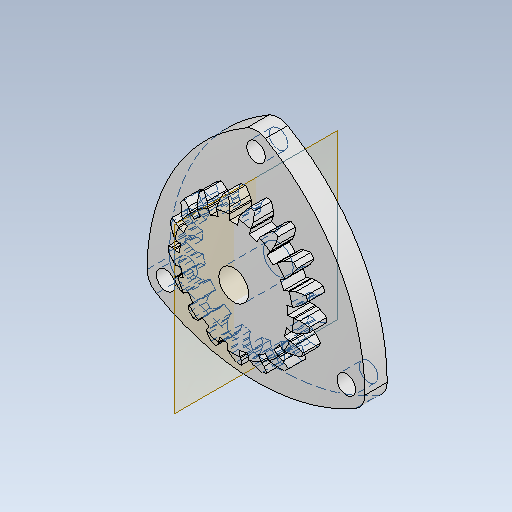
# Autodesk Inventor part: m1z17
Saved by Autodesk Inventor 2020 (Build 240168000, 168)
## iProperties
Created: 2020-10-28
Part Number: m1z17
Material: アルミニウム 2014-T4
Document SubType Name: Modeling
Designer: AA19065
Density: 2.8 g/cm^3
Appearance: サテン
Mass: 6.7317 g
Surface Area: 19.2727 cm^2
Volume: 2.40418 cm^3
Author: AA19065
Autodesk Inventor part; units mm, degrees
ref_plane "YZ Plane" through (0, 0, 0) normal (1, 0, 0) x (0, 1, 0)
ref_plane "XZ Plane" through (0, 0, 0) normal (0, 1, 0) x (-1, 0, 0)
ref_plane "XY Plane" through (0, 0, 0) normal (0, 0, 1) x (1, 0, 0)
sketch "スケッチ1" plane through (0, 0, 0) normal (0, 0, 1) x (1, 0, 0)
  arc A0 (149.1454, 113.0975) -> (149.1147, 112.9267) centre (149.977, 112.8598) ccw
  arc A1 (149.3297, 113.5561) -> (149.1454, 113.0975) centre (151.4433, 112.4406) ccw
  arc A2 (149.9133, 114.3943) -> (149.3297, 113.5561) centre (153.0232, 111.6068) ccw
  arc A3 (146.1768, 112.7838) -> (146.2098, 112.6135) centre (147.038, 112.8626) ccw
  arc A4 (146.1829, 113.2778) -> (146.1768, 112.7838) centre (148.5568, 113.0014) ccw
  arc A5 (146.4242, 114.2705) -> (146.1829, 113.2778) centre (150.3312, 112.7948) ccw
  arc A6 (143.5218, 111.419) -> (143.6141, 111.2721) centre (144.2964, 111.8035) ccw
  arc A7 (143.3491, 111.8818) -> (143.5218, 111.419) centre (145.6625, 112.4816) ccw
  arc A8 (143.2155, 112.8946) -> (143.3491, 111.8818) centre (147.3917, 112.93) ccw
  arc A9 (141.5392, 109.1872) -> (141.6783, 109.0836) centre (142.1226, 109.8256) ccw
  arc A10 (141.2109, 109.5563) -> (141.5392, 109.1872) centre (143.1514, 110.9514) ccw
  arc A11 (140.7205, 110.4525) -> (141.2109, 109.5563) centre (144.6019, 111.9941) ccw
  arc A12 (140.4967, 106.3899) -> (140.6638, 106.3435) centre (140.8101, 107.1959) ccw
  arc A13 (140.0572, 106.6155) -> (140.4967, 106.3899) centre (141.3627, 108.6174) ccw
  arc A14 (139.2762, 107.274) -> (140.0572, 106.6155) centre (142.3386, 110.1136) ccw
  arc A15 (140.535, 103.4049) -> (140.7076, 103.4221) centre (140.5361, 104.2697) ccw
  arc A16 (140.0437, 103.4565) -> (140.535, 103.4049) centre (140.538, 105.7948) ccw
  arc A17 (139.0776, 103.7885) -> (140.0437, 103.4565) centre (140.9074, 107.5426) ccw
  arc A18 (141.6491, 100.6353) -> (141.8039, 100.7137) centre (141.3377, 101.4421) ccw
  arc A19 (141.1723, 100.506) -> (141.6491, 100.6353) centre (140.7885, 102.8649) ccw
  arc A20 (140.1515, 100.4665) -> (141.1723, 100.506) centre (140.5016, 104.6281) ccw
  arc A21 (143.6884, 98.4552) -> (143.8044, 98.5842) centre (143.1066, 99.0951) ccw
  arc A22 (143.2906, 98.1624) -> (143.6884, 98.4552) centre (142.0805, 100.2234) ccw
  arc A23 (142.3529, 97.7568) -> (143.2906, 98.1624) centre (141.1761, 101.7639) ccw
  arc A24 (146.3776, 97.159) -> (146.4392, 97.3212) centre (145.6039, 97.5455) ccw
  arc A25 (146.1124, 96.7423) -> (146.3776, 97.159) centre (144.2395, 98.2269) ccw
  arc A26 (145.3846, 96.0254) -> (146.1124, 96.7423) centre (142.8397, 99.3367) ccw
  arc A27 (149.3534, 96.9218) -> (149.3522, 97.0953) centre (148.4924, 97.0027) ccw
  arc A28 (149.2566, 96.4374) -> (149.3534, 96.9218) centre (146.9739, 97.1453) ccw
  arc A29 (148.837, 95.506) -> (149.2566, 96.4374) centre (145.2677, 97.6744) ccw
  arc A30 (152.214, 97.7756) -> (152.1502, 97.9369) centre (151.3818, 97.54) ccw
  arc A31 (152.2987, 97.2889) -> (152.214, 97.7756) centre (149.9145, 97.1244) ccw
  arc A32 (152.2439, 96.2688) -> (152.2987, 97.2889) centre (148.1323, 97.0014) ccw
  arc A33 (154.5729, 99.6051) -> (154.4552, 99.7325) centre (153.8821, 99.0848) ccw
  arc A34 (154.8278, 99.1819) -> (154.5729, 99.6051) centre (152.6639, 98.1672) ccw
  arc A35 (155.1451, 98.2108) -> (154.8278, 99.1819) centre (151.0466, 97.4087) ccw
  arc A36 (156.1117, 102.1632) -> (155.9559, 102.2394) centre (155.6555, 101.4284) ccw
  arc A37 (156.5022, 101.8606) -> (156.1117, 102.1632) centre (154.8511, 100.1328) ccw
  arc A38 (157.1489, 101.0698) -> (156.5022, 101.8606) centre (153.6169, 98.8413) ccw
  arc A39 (156.6225, 105.1044) -> (156.4496, 105.1192) centre (156.4625, 104.2545) ccw
  arc A40 (157.0959, 104.9633) -> (156.6225, 105.1044) centre (156.1804, 102.7557) ccw
  arc A41 (157.9846, 104.4595) -> (157.0959, 104.9633) centre (155.4961, 101.1056) ccw
  arc A42 (156.0363, 108.0315) -> (155.8697, 107.9829) centre (156.1941, 107.1812) ccw
  arc A43 (156.5287, 108.071) -> (156.0363, 108.0315) centre (156.4725, 105.6818) ccw
  arc A44 (157.5394, 107.9223) -> (156.5287, 108.071) centre (156.4305, 103.8959) ccw
  arc A45 (154.4322, 110.5492) -> (154.2945, 110.4437) centre (154.8866, 109.8134) ccw
  arc A46 (154.8771, 110.7639) -> (154.4322, 110.5492) centre (155.6879, 108.5157) ccw
  arc A47 (155.8733, 110.9903) -> (154.8771, 110.7639) centre (156.2939, 106.8353) ccw
  arc A48 (152.027, 112.3175) -> (151.9367, 112.1693) centre (152.7165, 111.7954) ccw
  arc A49 (152.3643, 112.6784) -> (152.027, 112.3175) centre (153.9325, 110.8749) ccw
  arc A50 (153.2115, 113.2494) -> (152.3643, 112.6784) centre (155.1046, 109.5268) ccw
  arc A51 (147.8852, 112.9267) -> (147.8545, 113.0974) centre (147.023, 112.8598) ccw
  arc A52 (147.8545, 113.0974) -> (147.6704, 113.5559) centre (145.5566, 112.4406) ccw
  arc A53 (147.6704, 113.5559) -> (147.0867, 114.3943) centre (143.9767, 111.607) ccw
  arc A54 (145.0633, 112.1693) -> (144.973, 112.3175) centre (144.2835, 111.7954) ccw
  arc A55 (144.973, 112.3175) -> (144.6357, 112.6784) centre (143.0675, 110.8749) ccw
  arc A56 (144.6357, 112.6784) -> (143.7885, 113.2494) centre (141.8954, 109.5268) ccw
  arc A57 (142.7055, 110.4437) -> (142.5678, 110.5492) centre (142.1134, 109.8134) ccw
  arc A58 (142.5678, 110.5492) -> (142.1229, 110.7639) centre (141.3121, 108.5157) ccw
  arc A59 (142.1229, 110.7639) -> (141.1267, 110.9903) centre (140.7061, 106.8353) ccw
  arc A60 (141.1303, 107.9829) -> (140.9637, 108.0315) centre (140.8059, 107.1812) ccw
  arc A61 (140.9637, 108.0315) -> (140.4713, 108.071) centre (140.5275, 105.6818) ccw
  arc A62 (140.4713, 108.071) -> (139.4606, 107.9223) centre (140.5695, 103.8959) ccw
  arc A63 (140.5504, 105.1192) -> (140.3775, 105.1044) centre (140.5375, 104.2545) ccw
  arc A64 (140.3775, 105.1044) -> (139.9041, 104.9633) centre (140.8196, 102.7557) ccw
  arc A65 (139.9041, 104.9633) -> (139.0154, 104.4595) centre (141.5039, 101.1056) ccw
  arc A66 (141.0441, 102.2394) -> (140.8883, 102.1632) centre (141.3445, 101.4284) ccw
  arc A67 (140.8883, 102.1632) -> (140.4978, 101.8606) centre (142.1489, 100.1328) ccw
  arc A68 (140.4978, 101.8606) -> (139.8511, 101.0698) centre (143.3831, 98.8413) ccw
  arc A69 (142.5448, 99.7325) -> (142.4271, 99.6051) centre (143.1179, 99.0848) ccw
  arc A70 (142.4271, 99.6051) -> (142.1722, 99.1819) centre (144.3361, 98.1672) ccw
  arc A71 (142.1722, 99.1819) -> (141.8549, 98.2108) centre (145.9534, 97.4087) ccw
  arc A72 (144.8498, 97.9369) -> (144.786, 97.7756) centre (145.6182, 97.54) ccw
  arc A73 (144.786, 97.7756) -> (144.7013, 97.2889) centre (147.0855, 97.1244) ccw
  arc A74 (144.7013, 97.2889) -> (144.7561, 96.2688) centre (148.8677, 97.0014) ccw
  arc A75 (147.6478, 97.0953) -> (147.6466, 96.9218) centre (148.5076, 97.0027) ccw
  arc A76 (147.6466, 96.9218) -> (147.7434, 96.4374) centre (150.0261, 97.1453) ccw
  arc A77 (147.7434, 96.4374) -> (148.163, 95.506) centre (151.7323, 97.6744) ccw
  arc A78 (150.5608, 97.3212) -> (150.6224, 97.159) centre (151.3961, 97.5455) ccw
  arc A79 (150.6224, 97.159) -> (150.8876, 96.7423) centre (152.7605, 98.2269) ccw
  arc A80 (150.8876, 96.7423) -> (151.6154, 96.0254) centre (154.1603, 99.3367) ccw
  arc A81 (153.1956, 98.5842) -> (153.3116, 98.4552) centre (153.8934, 99.0951) ccw
  arc A82 (153.3116, 98.4552) -> (153.7094, 98.1624) centre (154.9195, 100.2234) ccw
  arc A83 (153.7094, 98.1624) -> (154.6471, 97.7568) centre (155.8239, 101.7639) ccw
  arc A84 (155.1961, 100.7137) -> (155.3509, 100.6353) centre (155.6623, 101.4421) ccw
  arc A85 (155.3509, 100.6353) -> (155.8277, 100.506) centre (156.2115, 102.8649) ccw
  arc A86 (155.8277, 100.506) -> (156.8485, 100.4665) centre (156.4984, 104.6281) ccw
  arc A87 (156.2924, 103.4221) -> (156.465, 103.4049) centre (156.4639, 104.2697) ccw
  arc A88 (156.465, 103.4049) -> (156.9563, 103.4565) centre (156.462, 105.7948) ccw
  arc A89 (156.9563, 103.4565) -> (157.9224, 103.7885) centre (156.0926, 107.5426) ccw
  arc A90 (156.3362, 106.3435) -> (156.5033, 106.3899) centre (156.1899, 107.1959) ccw
  arc A91 (156.5033, 106.3899) -> (156.9428, 106.6155) centre (155.6373, 108.6174) ccw
  arc A92 (156.9428, 106.6155) -> (157.7238, 107.274) centre (154.6614, 110.1136) ccw
  arc A93 (155.3217, 109.0836) -> (155.4608, 109.1872) centre (154.8774, 109.8256) ccw
  arc A94 (155.4608, 109.1872) -> (155.7891, 109.5563) centre (153.8486, 110.9514) ccw
  arc A95 (155.7891, 109.5563) -> (156.2795, 110.4525) centre (152.3981, 111.9941) ccw
  arc A96 (153.3859, 111.2721) -> (153.4782, 111.419) centre (152.7036, 111.8035) ccw
  arc A97 (153.4782, 111.419) -> (153.6509, 111.8818) centre (151.3375, 112.4816) ccw
  arc A98 (153.6509, 111.8818) -> (153.7845, 112.8946) centre (149.6083, 112.93) ccw
  arc A99 (150.7902, 112.6135) -> (150.8232, 112.7838) centre (149.962, 112.8626) ccw
  arc A100 (150.8232, 112.7838) -> (150.8171, 113.2778) centre (148.4432, 113.0014) ccw
  arc A101 (150.8171, 113.2778) -> (150.5758, 114.2705) centre (146.6688, 112.7948) ccw
  arc A102 (149.0605, 112.2283) -> (147.9394, 112.2283) centre (148.5, 105) ccw
  arc A103 (146.4115, 111.9427) -> (145.3661, 111.5377) centre (148.5, 105) ccw
  arc A104 (144.0446, 110.7194) -> (143.2161, 109.9641) centre (148.5, 105) ccw
  arc A105 (142.2793, 108.7237) -> (141.7796, 107.7201) centre (148.5, 105) ccw
  arc A106 (141.3543, 106.2251) -> (141.2508, 105.1088) centre (148.5, 105) ccw
  arc A107 (141.3942, 103.561) -> (141.701, 102.4827) centre (148.5, 105) ccw
  arc A108 (142.3939, 101.0913) -> (143.0695, 100.1966) centre (148.5, 105) ccw
  arc A109 (144.2182, 99.1495) -> (145.1714, 98.5593) centre (148.5, 105) ccw
  arc A110 (146.6208, 97.9978) -> (147.7228, 97.7918) centre (148.5, 105) ccw
  arc A111 (149.2772, 97.7918) -> (150.3792, 97.9978) centre (148.5, 105) ccw
  arc A112 (151.8286, 98.5593) -> (152.7818, 99.1495) centre (148.5, 105) ccw
  arc A113 (153.9305, 100.1966) -> (154.6061, 101.0913) centre (148.5, 105) ccw
  arc A114 (155.299, 102.4827) -> (155.6058, 103.561) centre (148.5, 105) ccw
  arc A115 (155.7492, 105.1088) -> (155.6457, 106.2251) centre (148.5, 105) ccw
  arc A116 (155.2204, 107.7201) -> (154.7207, 108.7237) centre (148.5, 105) ccw
  arc A117 (153.7839, 109.9641) -> (152.9554, 110.7194) centre (148.5, 105) ccw
  arc A118 (151.6339, 111.5377) -> (150.5885, 111.9427) centre (148.5, 105) ccw
  arc A119 (147.0867, 114.3943) -> (146.4242, 114.2705) centre (148.5, 105) ccw
  arc A120 (143.7885, 113.2494) -> (143.2155, 112.8946) centre (148.5, 105) ccw
  arc A121 (141.1267, 110.9903) -> (140.7205, 110.4525) centre (148.5, 105) ccw
  arc A122 (139.4606, 107.9223) -> (139.2762, 107.274) centre (148.5, 105) ccw
  arc A123 (139.0154, 104.4595) -> (139.0776, 103.7885) centre (148.5, 105) ccw
  arc A124 (139.8511, 101.0698) -> (140.1515, 100.4665) centre (148.5, 105) ccw
  arc A125 (141.8549, 98.2108) -> (142.3529, 97.7568) centre (148.5, 105) ccw
  arc A126 (144.7561, 96.2688) -> (145.3846, 96.0254) centre (148.5, 105) ccw
  arc A127 (148.163, 95.506) -> (148.837, 95.506) centre (148.5, 105) ccw
  arc A128 (151.6154, 96.0254) -> (152.2439, 96.2688) centre (148.5, 105) ccw
  arc A129 (154.6471, 97.7568) -> (155.1451, 98.2108) centre (148.5, 105) ccw
  arc A130 (156.8485, 100.4665) -> (157.1489, 101.0698) centre (148.5, 105) ccw
  arc A131 (157.9224, 103.7885) -> (157.9846, 104.4595) centre (148.5, 105) ccw
  arc A132 (157.7238, 107.274) -> (157.5394, 107.9223) centre (148.5, 105) ccw
  arc A133 (156.2795, 110.4525) -> (155.8733, 110.9903) centre (148.5, 105) ccw
  arc A134 (153.7845, 112.8946) -> (153.2115, 113.2494) centre (148.5, 105) ccw
  arc A135 (150.5758, 114.2705) -> (149.9133, 114.3943) centre (148.5, 105) ccw
  line L0 (149.0605, 112.2283) -> (149.1147, 112.9267)
  line L1 (146.4115, 111.9427) -> (146.2098, 112.6135)
  line L2 (144.0446, 110.7194) -> (143.6141, 111.2721)
  line L3 (142.2793, 108.7237) -> (141.6783, 109.0836)
  line L4 (141.3543, 106.2251) -> (140.6638, 106.3435)
  line L5 (141.3942, 103.561) -> (140.7076, 103.4221)
  line L6 (142.3939, 101.0913) -> (141.8039, 100.7137)
  line L7 (144.2182, 99.1495) -> (143.8044, 98.5842)
  line L8 (146.6208, 97.9978) -> (146.4392, 97.3212)
  line L9 (149.2772, 97.7918) -> (149.3522, 97.0953)
  line L10 (151.8286, 98.5593) -> (152.1502, 97.9369)
  line L11 (153.9305, 100.1966) -> (154.4552, 99.7325)
  line L12 (155.299, 102.4827) -> (155.9559, 102.2394)
  line L13 (155.7492, 105.1088) -> (156.4496, 105.1192)
  line L14 (155.2204, 107.7201) -> (155.8697, 107.9829)
  line L15 (153.7839, 109.9641) -> (154.2945, 110.4437)
  line L16 (151.6339, 111.5377) -> (151.9367, 112.1693)
  line L17 (147.9394, 112.2283) -> (147.8852, 112.9267)
  line L18 (145.3661, 111.5377) -> (145.0633, 112.1693)
  line L19 (143.2161, 109.9641) -> (142.7055, 110.4437)
  line L20 (141.7796, 107.7201) -> (141.1303, 107.9829)
  line L21 (141.2508, 105.1088) -> (140.5504, 105.1192)
  line L22 (141.701, 102.4827) -> (141.0441, 102.2394)
  line L23 (143.0695, 100.1966) -> (142.5448, 99.7325)
  line L24 (145.1714, 98.5593) -> (144.8498, 97.9369)
  line L25 (147.7228, 97.7918) -> (147.6478, 97.0953)
  line L26 (150.3792, 97.9978) -> (150.5608, 97.3212)
  line L27 (152.7818, 99.1495) -> (153.1956, 98.5842)
  line L28 (154.6061, 101.0913) -> (155.1961, 100.7137)
  line L29 (155.6058, 103.561) -> (156.2924, 103.4221)
  line L30 (155.6457, 106.2251) -> (156.3362, 106.3435)
  line L31 (154.7207, 108.7237) -> (155.3217, 109.0836)
  line L32 (152.9554, 110.7194) -> (153.3859, 111.2721)
  line L33 (150.5885, 111.9427) -> (150.7902, 112.6135)
  line L34 (137, 105) -> (160, 105)
  line L35 (148.5, 93.5) -> (148.5, 116.5)
  line L36 (178, 114.5) -> (248, 114.5)
  line L37 (178, 106.5) -> (248, 106.5)
  line L38 (178, 98.5) -> (248, 98.5)
  line L39 (178, 90.5) -> (248, 90.5)
  line L40 (178, 82.5) -> (248, 82.5)
  line L41 (178, 74.5) -> (248, 74.5)
  line L42 (178, 66.5) -> (248, 66.5)
  line L43 (178, 58.5) -> (248, 58.5)
  line L44 (178, 50.5) -> (248, 50.5)
  line L45 (178, 42.5) -> (248, 42.5)
  line L46 (178, 34.5) -> (248, 34.5)
  line L47 (178, 26.5) -> (248, 26.5)
  line L48 (178, 18.5) -> (248, 18.5)
  line L49 (178, 114.5) -> (178, 18.5)
  line L50 (248, 114.5) -> (248, 18.5)
  line L51 (213, 106.5) -> (213, 18.5)
  circle A136 centre (148.5, 105) radius 2
  circle A137 centre (148.5, 119) radius 1.25
  circle A138 centre (136.3756, 98) radius 1.25
  circle A139 centre (160.6244, 98) radius 1.25
  circle A140 centre (148.5, 119) radius 2.5
  circle A141 centre (136.3756, 98) radius 2.5
  circle A142 centre (160.6244, 98) radius 2.5
  arc A143 (147.25, 121.1651) -> (133.8756, 98) centre (160.6244, 98) ccw
  arc A144 (135.1256, 95.8349) -> (161.8744, 95.8349) centre (148.5, 119) ccw
  arc A145 (163.1244, 98) -> (149.75, 121.1651) centre (136.3756, 98) ccw
  point P0 (0, 0)
  point P1 (184, 108.5)
  point P2 (186.5, 100.5)
  point P3 (186.5, 92.5)
  point P4 (184, 84.5)
  point P5 (186.5, 76.5)
  point P6 (181.5, 68.5)
  point P7 (184, 60.5)
  point P8 (184, 52.5)
  point P9 (184, 44.5)
  point P10 (186.5, 36.5)
  point P11 (186.5, 28.5)
  point P12 (184, 20.5)
  point P13 (214, 100.5)
  point P14 (229, 92.5)
  point P15 (230.25, 84.5)
  point P16 (226.5, 76.5)
  point P17 (229, 68.5)
  point P18 (222.75, 60.5)
  point P19 (229, 52.5)
  point P20 (226.5, 44.5)
  point P21 (224, 36.5)
  point P22 (231.5, 28.5)
  point P23 (231.5, 20.5)
  point P24 (149.5, 130)
  point P25 (149.5, 124)
  point P26 (166.75, 130)
  point P27 (167.8125, 124)
  dimension "d0" = 4
  dimension "d1" = 2.5
  dimension "d2" = 14
  dimension "d5" = 360
  dimension "d7" = 5
  dimension "d10" = 360
  constraints: 216 point on circle, 112 centre point, 105 equal radius, 105 tangent, 100 end point, 20 horizontal, 13 parallel, 4 coincident, 3 horizontal alignment, 2 midpoint, 2 perpendicular, 1 point on line, 1 vertical, 569 other
  measures "d0" diameter of A136
  measures "d1" diameter of A137
  measures "d2" distance of A136.centre A137.centre
  measures "d7" diameter of A140
extrude "押し出し1" add sketch "スケッチ1" along normal blind 3 contours A1 A2 A135 A101 A100 A99 L33 A118 L16 A48 A49 A50 A134 A98 A97 A96 L32 A117 L15 A45 A46 A47 A133 A95 A94 A93 L31 A116 L14 A42 A43 A44 A132 A92 A91 A90 L30 A115 L13 A39 A40 L34 A136 L35 A102 L0 A0 | L35 A136 L34 A64 A63 L21 A106 L4 A12 A13 A14 A122 A62 A61 A60 L20 A105 L3 A9 A10 A11 A121 A59 A58 A57 L19 A104 L2 A6 A7 A8 A120 A56 A55 A54 L18 A103 L1 A3 A4 A5 A119 A53 A52 A51 L17 A102 | L34 A40 A41 A131 A89 A88 A87 L29 A114 L12 A36 A37 A38 A130 A86 A85 A84 L28 A113 L11 A33 A34 A35 A129 A83 A82 A81 L27 A112 L10 A30 A31 A32 A128 A80 A79 A78 L26 A111 L9 A27 A28 A29 A127 L35 A136 | A136 L35 A127 A77 A76 A75 L25 A110 L8 A24 A25 A26 A126 A74 A73 A72 L24 A109 L7 A21 A22 A23 A125 A71 A70 A69 L23 A108 L6 A18 A19 A20 A124 A68 A67 A66 L22 A107 L5 A15 A16 A17 A123 A65 A64 L34
extrude "押し出し2" add sketch "スケッチ1" against normal blind 3 contours A1 A2 A135 A101 A100 A99 L33 A118 L16 A48 A49 A50 A134 A98 A97 A96 L32 A117 L15 A45 A46 A47 A133 A95 A94 A93 L31 A116 L14 A42 A43 A44 A132 A92 A91 A90 L30 A115 L13 A39 A40 L34 A136 L35 A102 L0 A0 | L35 A136 L34 A64 A63 L21 A106 L4 A12 A13 A14 A122 A62 A61 A60 L20 A105 L3 A9 A10 A11 A121 A59 A58 A57 L19 A104 L2 A6 A7 A8 A120 A56 A55 A54 L18 A103 L1 A3 A4 A5 A119 A53 A52 A51 L17 A102 | L34 A40 A41 A131 A89 A88 A87 L29 A114 L12 A36 A37 A38 A130 A86 A85 A84 L28 A113 L11 A33 A34 A35 A129 A83 A82 A81 L27 A112 L10 A30 A31 A32 A128 A80 A79 A78 L26 A111 L9 A27 A28 A29 A127 L35 A136 | A136 L35 A127 A77 A76 A75 L25 A110 L8 A24 A25 A26 A126 A74 A73 A72 L24 A109 L7 A21 A22 A23 A125 A71 A70 A69 L23 A108 L6 A18 A19 A20 A124 A68 A67 A66 L22 A107 L5 A15 A16 A17 A123 A65 A64 L34 | A140 | A140 A145 A142 A144 A141 A143 | A142 | A141
ref_plane "作業平面1" through (148.5, 105, 0) normal (1, 0, 0) x (0, 1, 0)
sketch "スケッチ2" plane through (148.5, 105, 0) normal (1, 0, 0) x (0, 1, 0)
  line L0 (0, 10.3213) -> (0, -13.9718)
  line L1 (-9.494, 3) -> (-9.5, 3) projected
  line L2 (-9.5, 0) -> (-9.5, 3) projected
  line L3 (2.7201, 3) -> (3.7237, 3) projected
  line L4 (3.7237, 3) -> (4.0836, 3) projected
  line L5 (4.0836, 3) -> (4.1872, 3) projected
  line L6 (4.1872, 3) -> (4.5563, 3) projected
  line L7 (4.5563, 3) -> (5.4525, 3) projected
  line L8 (5.4525, 3) -> (5.9903, 3) projected
  line L9 (5.9903, 3) -> (5.7639, 3) projected
  line L10 (5.7639, 3) -> (5.5492, 3) projected
  line L11 (5.5492, 3) -> (5.4437, 3) projected
  line L12 (5.4437, 3) -> (4.9641, 3) projected
  line L13 (4.9641, 3) -> (5.7194, 3) projected
  line L14 (5.7194, 3) -> (6.2721, 3) projected
  line L15 (6.2721, 3) -> (6.419, 3) projected
  line L16 (6.419, 3) -> (6.8818, 3) projected
  line L17 (6.8818, 3) -> (7.8946, 3) projected
  line L18 (7.8946, 3) -> (8.2494, 3) projected
  line L19 (8.2494, 3) -> (7.6784, 3) projected
  line L20 (7.6784, 3) -> (7.3175, 3) projected
  line L21 (7.3175, 3) -> (7.1693, 3) projected
  line L22 (7.1693, 3) -> (6.5377, 3) projected
  line L23 (6.5377, 3) -> (6.9427, 3) projected
  line L24 (6.9427, 3) -> (7.6135, 3) projected
  line L25 (7.6135, 3) -> (7.7838, 3) projected
  line L26 (7.7838, 3) -> (8.2778, 3) projected
  line L27 (8.2778, 3) -> (9.2705, 3) projected
  line L28 (9.2705, 3) -> (9.3943, 3) projected
  line L29 (9.3943, 3) -> (8.5561, 3) projected
  line L30 (8.5561, 3) -> (8.0975, 3) projected
  line L31 (8.0975, 3) -> (7.9267, 3) projected
  line L32 (7.9267, 3) -> (7.2283, 3) projected
  line L33 (7.2283, 3) -> (7.2283, 3) projected
  line L34 (7.2283, 3) -> (7.9267, 3) projected
  line L35 (7.9267, 3) -> (8.0974, 3) projected
  line L36 (8.0974, 3) -> (8.5559, 3) projected
  line L37 (8.5559, 3) -> (9.3943, 3) projected
  line L38 (9.3943, 3) -> (9.2705, 3) projected
  line L39 (9.2705, 3) -> (8.2778, 3) projected
  line L40 (8.2778, 3) -> (7.7838, 3) projected
  line L41 (7.7838, 3) -> (7.6135, 3) projected
  line L42 (7.6135, 3) -> (6.9427, 3) projected
  line L43 (6.9427, 3) -> (6.5377, 3) projected
  line L44 (6.5377, 3) -> (7.1693, 3) projected
  line L45 (7.1693, 3) -> (7.3175, 3) projected
  line L46 (7.3175, 3) -> (7.6784, 3) projected
  line L47 (7.6784, 3) -> (8.2494, 3) projected
  line L48 (8.2494, 3) -> (7.8946, 3) projected
  line L49 (7.8946, 3) -> (6.8818, 3) projected
  line L50 (6.8818, 3) -> (6.419, 3) projected
  line L51 (6.419, 3) -> (6.2721, 3) projected
  line L52 (6.2721, 3) -> (5.7194, 3) projected
  line L53 (5.7194, 3) -> (4.9641, 3) projected
  line L54 (4.9641, 3) -> (5.4437, 3) projected
  line L55 (5.4437, 3) -> (5.5492, 3) projected
  line L56 (5.5492, 3) -> (5.7639, 3) projected
  line L57 (5.7639, 3) -> (5.9903, 3) projected
  line L58 (5.9903, 3) -> (5.4525, 3) projected
  line L59 (5.4525, 3) -> (4.5563, 3) projected
  line L60 (4.5563, 3) -> (4.1872, 3) projected
  line L61 (4.1872, 3) -> (4.0836, 3) projected
  line L62 (4.0836, 3) -> (3.7237, 3) projected
  line L63 (3.7237, 3) -> (2.7201, 3) projected
  line L64 (2.7201, 3) -> (2.9829, 3) projected
  line L65 (2.9829, 3) -> (3.0315, 3) projected
  line L66 (3.0315, 3) -> (3.071, 3) projected
  line L67 (3.071, 3) -> (2.9223, 3) projected
  line L68 (2.9223, 3) -> (2.274, 3) projected
  line L69 (2.274, 3) -> (1.6155, 3) projected
  line L70 (1.6155, 3) -> (1.3899, 3) projected
  line L71 (1.3899, 3) -> (1.3435, 3) projected
  line L72 (1.3435, 3) -> (1.2251, 3) projected
  line L73 (1.2251, 3) -> (0.1088, 3) projected
  line L74 (0.1088, 3) -> (0.1192, 3) projected
  line L75 (0.1192, 3) -> (0.1044, 3) projected
  line L76 (0.1044, 3) -> (-0.0367, 3) projected
  line L77 (-0.0367, 3) -> (-0.5405, 3) projected
  line L78 (-0.5405, 3) -> (-1.2115, 3) projected
  line L79 (-1.2115, 3) -> (-1.5435, 3) projected
  line L80 (-1.5435, 3) -> (-1.5951, 3) projected
  line L81 (-1.5951, 3) -> (-1.5779, 3) projected
  line L82 (-1.5779, 3) -> (-1.439, 3) projected
  line L83 (-1.439, 3) -> (-2.5173, 3) projected
  line L84 (-2.5173, 3) -> (-2.7606, 3) projected
  line L85 (-2.7606, 3) -> (-2.8368, 3) projected
  line L86 (-2.8368, 3) -> (-3.1394, 3) projected
  line L87 (-3.1394, 3) -> (-3.9302, 3) projected
  line L88 (-3.9302, 3) -> (-4.5335, 3) projected
  line L89 (-4.5335, 3) -> (-4.494, 3) projected
  line L90 (-4.494, 3) -> (-4.3647, 3) projected
  line L91 (-4.3647, 3) -> (-4.2863, 3) projected
  line L92 (-4.2863, 3) -> (-3.9087, 3) projected
  line L93 (-3.9087, 3) -> (-4.8034, 3) projected
  line L94 (-4.8034, 3) -> (-5.2675, 3) projected
  line L95 (-5.2675, 3) -> (-5.3949, 3) projected
  line L96 (-5.3949, 3) -> (-5.8181, 3) projected
  line L97 (-5.8181, 3) -> (-6.7892, 3) projected
  line L98 (-6.7892, 3) -> (-7.2432, 3) projected
  line L99 (-7.2432, 3) -> (-6.8376, 3) projected
  line L100 (-6.8376, 3) -> (-6.5448, 3) projected
  line L101 (-6.5448, 3) -> (-6.4158, 3) projected
  line L102 (-6.4158, 3) -> (-5.8505, 3) projected
  line L103 (-5.8505, 3) -> (-6.4407, 3) projected
  line L104 (-6.4407, 3) -> (-7.0631, 3) projected
  line L105 (-7.0631, 3) -> (-7.2244, 3) projected
  line L106 (-7.2244, 3) -> (-7.7111, 3) projected
  line L107 (-7.7111, 3) -> (-8.7312, 3) projected
  line L108 (-8.7312, 3) -> (-8.9746, 3) projected
  line L109 (-8.9746, 3) -> (-8.2577, 3) projected
  line L110 (-8.2577, 3) -> (-7.841, 3) projected
  line L111 (-7.841, 3) -> (-7.6788, 3) projected
  line L112 (-7.6788, 3) -> (-7.0022, 3) projected
  line L113 (-7.0022, 3) -> (-7.2082, 3) projected
  line L114 (-7.2082, 3) -> (-7.9047, 3) projected
  line L115 (-7.9047, 3) -> (-8.0782, 3) projected
  line L116 (-8.0782, 3) -> (-8.5626, 3) projected
  line L117 (-8.5626, 3) -> (-9.494, 3) projected
  line L118 (-9.494, 3) -> (-9.494, 3) projected
  line L119 (-9.494, 3) -> (-8.5626, 3) projected
  line L120 (-8.5626, 3) -> (-8.0782, 3) projected
  line L121 (-8.0782, 3) -> (-7.9047, 3) projected
  line L122 (-7.9047, 3) -> (-7.2082, 3) projected
  line L123 (-7.2082, 3) -> (-7.0022, 3) projected
  line L124 (-7.0022, 3) -> (-7.6788, 3) projected
  line L125 (-7.6788, 3) -> (-7.841, 3) projected
  line L126 (-7.841, 3) -> (-8.2577, 3) projected
  line L127 (-8.2577, 3) -> (-8.9746, 3) projected
  line L128 (-8.9746, 3) -> (-8.7312, 3) projected
  line L129 (-8.7312, 3) -> (-7.7111, 3) projected
  line L130 (-7.7111, 3) -> (-7.2244, 3) projected
  line L131 (-7.2244, 3) -> (-7.0631, 3) projected
  line L132 (-7.0631, 3) -> (-6.4407, 3) projected
  line L133 (-6.4407, 3) -> (-5.8505, 3) projected
  line L134 (-5.8505, 3) -> (-6.4158, 3) projected
  line L135 (-6.4158, 3) -> (-6.5448, 3) projected
  line L136 (-6.5448, 3) -> (-6.8376, 3) projected
  line L137 (-6.8376, 3) -> (-7.2432, 3) projected
  line L138 (-7.2432, 3) -> (-6.7892, 3) projected
  line L139 (-6.7892, 3) -> (-5.8181, 3) projected
  line L140 (-5.8181, 3) -> (-5.3949, 3) projected
  line L141 (-5.3949, 3) -> (-5.2675, 3) projected
  line L142 (-5.2675, 3) -> (-4.8034, 3) projected
  line L143 (-4.8034, 3) -> (-3.9087, 3) projected
  line L144 (-3.9087, 3) -> (-4.2863, 3) projected
  line L145 (-4.2863, 3) -> (-4.3647, 3) projected
  line L146 (-4.3647, 3) -> (-4.494, 3) projected
  line L147 (-4.494, 3) -> (-4.5335, 3) projected
  line L148 (-4.5335, 3) -> (-3.9302, 3) projected
  line L149 (-3.9302, 3) -> (-3.1394, 3) projected
  line L150 (-3.1394, 3) -> (-2.8368, 3) projected
  line L151 (-2.8368, 3) -> (-2.7606, 3) projected
  line L152 (-2.7606, 3) -> (-2.5173, 3) projected
  line L153 (-2.5173, 3) -> (-1.439, 3) projected
  line L154 (-1.439, 3) -> (-1.5779, 3) projected
  line L155 (-1.5779, 3) -> (-1.5951, 3) projected
  line L156 (-1.5951, 3) -> (-1.5435, 3) projected
  line L157 (-1.5435, 3) -> (-1.2115, 3) projected
  line L158 (-1.2115, 3) -> (-0.5405, 3) projected
  line L159 (-0.5405, 3) -> (-0.0367, 3) projected
  line L160 (-0.0367, 3) -> (0.1044, 3) projected
  line L161 (0.1044, 3) -> (0.1192, 3) projected
  line L162 (0.1192, 3) -> (0.1088, 3) projected
  line L163 (0.1088, 3) -> (1.2251, 3) projected
  line L164 (1.2251, 3) -> (1.3435, 3) projected
  line L165 (1.3435, 3) -> (1.3899, 3) projected
  line L166 (1.3899, 3) -> (1.6155, 3) projected
  line L167 (1.6155, 3) -> (2.274, 3) projected
  line L168 (2.274, 3) -> (2.9223, 3) projected
  line L169 (2.9223, 3) -> (3.071, 3) projected
  line L170 (3.071, 3) -> (3.0315, 3) projected
  line L171 (3.0315, 3) -> (2.9829, 3) projected
  line L172 (2.9829, 3) -> (2.7201, 3) projected
  line L173 (-2, 3) -> (2, 3) projected
  line L174 (-9.5, 2.3) -> (-8, 3)
  point P0 (-105, 0)
  point P1 (0, 0)
  point P2 (0, 0)
  point P3 (0, 0)
  point P4 (-7.5, 3)
  point P5 (-8, 3)
  dimension "d16" = 1.5
  dimension "d17" = 0.7
  constraints: 4 end point, 3 point on line, 1 vertical
  measures "d16" distance of L2.end L174.end
  measures "d17" distance of L174.start L2.end
revolve "回転1" cut sketch "スケッチ2" angle 360 about axis through (148.5, 105, 10.3213) along (0, 0, -1)
